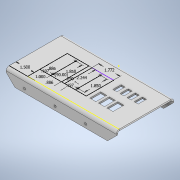
# Autodesk Inventor part: sheetmetalrightside
Saved by Autodesk Inventor 2020.2 (Build 242310000, 310)
## iProperties
Created: 2020-02-05
Part Number: sheetmetalrightside
Material: Generic
Document SubType Name: Sheet Metal
Designer: ColinP
Density: 1 g/cm^3
Sheet Metal Rule: Default
Appearance: Default
Author: ColinP
Autodesk Inventor part; units mm, degrees
ref_plane "YZ Plane" through (0, 0, 0) normal (1, 0, 0) x (0, 1, 0)
ref_plane "XZ Plane" through (0, 0, 0) normal (0, 1, 0) x (-1, 0, 0)
ref_plane "XY Plane" through (0, 0, 0) normal (0, 0, 1) x (1, 0, 0)
sketch "Sketch1" plane through (0, 0, 0) normal (0, 0, 1) x (1, 0, 0)
  line L0 (114.3, 63.5) -> (-114.3, 63.5)
  line L1 (-114.3, 63.5) -> (-114.3, -63.5)
  line L2 (-114.3, -63.5) -> (114.3, -63.5)
  line L3 (114.3, -63.5) -> (114.3, 63.5)
  point P0 (0, 0)
  dimension "d0" = 228.6
  dimension "d1" = 127
  measures "d0" distance of L2.end L1.end
  measures "d1" distance of L1.end L0.end
extrude "Plate1" add sketch "Sketch1" along normal blind 3.048
sketch "Sketch2" plane through (0, 0, 3.048) normal (0, 0, 1) x (1, 0, 0)
  line L0 (114.3, 63.5) -> (-114.3, 63.5)
  line L1 (-114.3, 63.5) -> (-96.3395, 81.4605)
  line L2 (-114.3, 63.5) -> (-88.9, 63.5) construction
  line L3 (114.3, 63.5) -> (96.3395, 81.4605)
  line L4 (114.3, 63.5) -> (139.7, 63.5) construction
  line L5 (96.3395, 81.4605) -> (-96.3395, 81.4605)
  line L6 (-114.3, 63.5) -> (-114.3, -63.5)
  line L7 (-114.3, -63.5) -> (-96.3395, -81.4605)
  line L8 (-114.3, -63.5) -> (-88.9, -63.5) construction
  line L9 (-96.3395, -81.4605) -> (96.3395, -81.4605)
  line L10 (-114.3, -63.5) -> (114.3, -63.5)
  line L11 (96.3395, -81.4605) -> (114.3, -63.5)
  point P0 (0, 0)
  dimension "d3" = 25.4
  dimension "d4" = 45
  dimension "d5" = 25.4
  dimension "d6" = 135
  dimension "d7" = 25.4
  dimension "d8" = 45
  measures "d3" distance of L0.end L1.end
  measures "d4" angle of L2 L1
  measures "d5" distance of L0.start L3.end
  measures "d6" angle of L4 L3
  measures "d7" distance of L6.end L7.end
  measures "d8" angle of L7 L8
sheet face with bend "Face2" sketch "Sketch2" thickness 3.048 toward (0, 0, -1) bend radius 3.048 relief straight relief width 3.048 relief depth 1.524
bend "Bend1"
sketch "Sketch3" plane through (0, 0, 3.048) normal (0, 0, 1) x (1, 0, 0)
  line L0 (-114.3, 63.5) -> (-114.3, -63.5) projected
  line L1 (-114.3, 63.5) -> (-114.3, 57.15)
  line L2 (-114.3, 57.15) -> (114.3, 57.15)
  line L3 (114.3, 63.5) -> (114.3, -63.5) projected
  line L4 (114.3, -63.5) -> (114.3, -57.15)
  line L5 (114.3, -57.15) -> (-114.3, -57.15)
  point P0 (0, 0)
  dimension "d14" = 6.35
  dimension "d15" = 6.35
  constraints: 8 end point, 4 point on line, 2 perpendicular
  measures "d14" distance of L0.start L1.end
  measures "d15" distance of L3.end L4.end
fold "Fold1" angle 90 bend radius 3.048 thickness 3.048 k factor 0.44 line from (-114.3, 57.15, 3.048) to (114.3, 57.15, 3.048) line at bend centre moving side (0, 1, 0) folds toward (0, 0, 1)
sketch "Sketch4" plane through (0, 0, 3.048) normal (0, 0, 1) x (1, 0, 0)
  line L0 (-114.3, -63.5) -> (-114.3, 53.7028) projected
  line L1 (-114.3, -63.5) -> (-114.3, -57.15)
  line L2 (-114.3, -57.15) -> (114.3, -57.15)
  line L3 (114.3, -63.5) -> (114.3, 53.7028) projected
  point P0 (0, 0)
  dimension "d22" = 6.35
  constraints: 4 end point, 2 point on line, 1 perpendicular
  measures "d22" distance of L0.start L1.end
fold "Fold2" angle 90 bend radius 3.048 thickness 3.048 k factor 0.44 line from (-114.3, -57.15, 3.048) to (114.3, -57.15, 3.048) line at bend centre moving side (0, 1, 0) folds toward (0, 0, 1)
sketch "Sketch5" plane through (-114.3, -54.5012, 113.5016) normal (0, 1, 0) x (1, 0, 0)
  line L0 (0, 0) -> (228.6, 0) projected
  line L1 (228.6, 0) -> (190.5, 0)
  line L2 (190.5, 0) -> (190.5, 25.4)
  line L3 (190.5, 25.4) -> (190.5, 48.006)
  line L4 (190.5, 48.006) -> (177.8, 48.006)
  line L5 (177.8, 48.006) -> (177.8, 25.4)
  line L6 (177.8, 25.4) -> (190.5, 25.4)
  line L7 (177.8, 48.006) -> (172.72, 48.006)
  line L8 (172.72, 48.006) -> (160.02, 48.006)
  line L9 (160.02, 48.006) -> (160.02, 25.4)
  line L10 (160.02, 25.4) -> (172.72, 25.4)
  line L11 (172.72, 25.4) -> (172.72, 48.006)
  line L12 (160.02, 48.006) -> (154.94, 48.006)
  line L13 (154.94, 48.006) -> (154.94, 25.4)
  line L14 (154.94, 25.4) -> (142.24, 25.4)
  line L15 (142.24, 25.4) -> (142.24, 48.006)
  line L16 (142.24, 48.006) -> (154.94, 48.006)
  line L17 (203.2, 107.4056) -> (203.2, 82.0056)
  line L18 (203.2, 107.4056) -> (228.6, 107.4056) construction
  line L19 (203.2, 82.0056) -> (194.818, 82.0056)
  line L20 (194.818, 82.0056) -> (194.818, 64.9876)
  line L21 (194.818, 64.9876) -> (203.2, 64.9876)
  line L22 (203.2, 64.9876) -> (203.2, 82.0056)
  line L23 (194.818, 82.0056) -> (188.468, 82.0056)
  line L24 (188.468, 82.0056) -> (180.086, 82.0056)
  line L25 (180.086, 82.0056) -> (180.086, 64.9876)
  line L26 (180.086, 64.9876) -> (188.468, 64.9876)
  line L27 (188.468, 64.9876) -> (188.468, 82.0056)
  line L28 (180.086, 82.0056) -> (173.736, 82.0056)
  line L29 (173.736, 82.0056) -> (173.736, 64.9876)
  line L30 (173.736, 64.9876) -> (165.354, 64.9876)
  line L31 (165.354, 64.9876) -> (165.354, 82.0056)
  line L32 (165.354, 82.0056) -> (173.736, 82.0056)
  line L33 (165.354, 82.0056) -> (159.004, 82.0056)
  line L34 (159.004, 82.0056) -> (159.004, 64.9876)
  line L35 (159.004, 64.9876) -> (150.622, 64.9876)
  line L36 (150.622, 64.9876) -> (150.622, 82.0056)
  line L37 (150.622, 82.0056) -> (159.004, 82.0056)
  line L38 (228.6, 0) -> (228.6, 107.4056) projected
  line L39 (203.2, 107.4056) -> (228.6, 107.4056)
  point P0 (114.3, 113.5016)
  dimension "d34" = 38.1
  dimension "d35" = 25.4
  dimension "d36" = 22.606
  dimension "d37" = 12.7
  dimension "d38" = 5.08
  dimension "d39" = 12.7
  dimension "d40" = 5.08
  dimension "d41" = 12.7
  dimension "d42" = 25.4
  dimension "d44" = 8.382
  dimension "d45" = 17.018
  dimension "d46" = 6.35
  dimension "d47" = 8.382
  dimension "d48" = 6.35
  dimension "d49" = 8.382
  dimension "d50" = 6.35
  dimension "d51" = 8.382
  dimension "d86" = 25.4
  constraints: 76 end point, 21 perpendicular, 14 point on line, 6 horizontal, 3 vertical, 1 collinear
  measures "d34" distance of L0.end L1.end
  measures "d35" distance of L1.end L2.end
  measures "d36" distance of L2.end L3.end
  measures "d37" distance of L3.end L4.end
  measures "d38" distance of L4.end L7.end
  measures "d39" distance of L7.end L8.end
  measures "d40" distance of L8.end L12.end
  measures "d41" distance of L13.end L14.end
  measures "d42" distance of L17.start L17.end
  measures "d44" distance of L17.end L19.end
  measures "d45" distance of L19.end L20.end
  measures "d46" distance of L19.end L23.end
  measures "d47" distance of L23.end L24.end
  measures "d48" distance of L24.end L28.end
  measures "d49" distance of L29.end L30.end
  measures "d50" distance of L31.end L33.end
  measures "d51" distance of L34.end L35.end
  measures "d86" distance of L17.start L18.end
extrude "Cut1" cut sketch "Sketch5" against normal blind 3.048
sketch "Sketch6" plane through (-114.3, -54.5012, 113.5016) normal (0, 1, 0) x (1, 0, 0)
  line L0 (0, 0) -> (228.6, 0) projected
  line L1 (0, 0) -> (38.1, 0)
  line L2 (38.1, 0) -> (38.1, 25.4)
  line L3 (38.1, 25.4) -> (60.6, 25.4)
  line L4 (60.6, 25.4) -> (83.1, 25.4)
  line L5 (83.1, 25.4) -> (83.1, 82.4)
  line L6 (83.1, 82.4) -> (38.1, 82.4)
  line L7 (38.1, 82.4) -> (38.1, 25.4)
  line L8 (60.6, 25.4) -> (60.6, 30.4)
  line L9 (60.6, 30.4) -> (60.6, 77.4)
  line L10 (83.1, 25.4) -> (89.45, 25.4)
  line L11 (89.45, 25.4) -> (89.45, 82.4)
  line L12 (89.45, 82.4) -> (134.45, 82.4)
  line L13 (134.45, 82.4) -> (134.45, 25.4)
  line L14 (134.45, 25.4) -> (89.45, 25.4)
  line L15 (111.95, 25.4) -> (111.95, 30.4)
  line L16 (111.95, 30.4) -> (111.95, 77.4)
  point P0 (114.3, 113.5016)
  dimension "d54" = 38.1
  dimension "d55" = 25.4
  dimension "d56" = 22.5
  dimension "d57" = 22.5
  dimension "d58" = 57
  dimension "d59" = 90
  dimension "d60" = 5
  dimension "d61" = 47
  dimension "d62" = 6.35
  dimension "d63" = 45
  dimension "d64" = 5
  dimension "d65" = 47
  constraints: 32 end point, 8 perpendicular, 5 point on line, 2 horizontal, 2 vertical, 1 midpoint
  measures "d54" distance of L0.start L1.end
  measures "d55" distance of L1.end L2.end
  measures "d56" distance of L2.end L3.end
  measures "d57" distance of L3.end L4.end
  measures "d58" distance of L4.end L5.end
  measures "d59" angle of L5 L4
  measures "d60" distance of L3.end L8.end
  measures "d61" distance of L8.end L9.end
  measures "d62" distance of L4.end L10.end
  measures "d63" distance of L11.end L12.end
  measures "d64" distance of L15.start L15.end
  measures "d65" distance of L15.end L16.end
hole "Hole1" at (-2.35, -54.5012, 83.1016) at (-2.35, -54.5012, 36.1016) at (-53.7, -54.5012, 36.1016) at (-53.7, -54.5012, 83.1016) direction (0, -1, 0) diameter 4.4958 depth 3.048 clearance for "Flat Head Machine Screw (82)" size "#8" standard "Ansi Unified Screw Threads"
sketch "Sketch7" plane through (96.3395, -81.4605, 119.5976) normal (0, 0, -1) x (-1, 0, 0)
  line L0 (-17.9605, 17.9605) -> (-17.9605, 20.8633) projected
  line L1 (-17.9605, 17.9605) -> (-17.9605, 7.8005)
  line L2 (-17.9605, 7.8005) -> (210.6395, 7.8005)
  line L3 (-17.9605, 7.8005) -> (45.5395, 7.8005)
  line L4 (45.5395, 7.8005) -> (109.0395, 7.8005)
  line L5 (109.0395, 7.8005) -> (172.5395, 7.8005)
  point P0 (96.3395, 81.4605)
  dimension "d73" = 10.16
  dimension "d74" = 228.6
  dimension "d75" = 90
  dimension "d76" = 63.5
  dimension "d77" = 63.5
  dimension "d78" = 63.5
  constraints: 10 end point, 3 point on line, 1 perpendicular, 1 vertical
  measures "d73" distance of L0.start L1.end
  measures "d74" distance of L1.end L2.end
  measures "d75" angle of L2 L1
  measures "d76" distance of L1.end L3.end
  measures "d77" distance of L3.end L4.end
  measures "d78" distance of L4.end L5.end
hole "Hole2" at (50.8, -73.66, 119.5976) at (-12.7, -73.66, 119.5976) at (-76.2, -73.66, 119.5976) direction (0, 0, -1) diameter 4.4958 depth 3.048 clearance for "Flat Head Machine Screw (82)" size "#8" standard "Ansi Unified Screw Threads"
equation "\"d2\" = Thickness"
equation "\"d16\" = BendReliefWidth"
equation "\"d17\" = BendReliefDepth"
equation "\"d18\" = MinimumRemnant"
equation "\"d19\" = TransitionRadius"
equation "\"d21\" = BendRadius"
equation "\"d23\" = BendReliefWidth"
equation "\"d24\" = BendReliefDepth"
equation "\"d25\" = MinimumRemnant"
equation "\"d26\" = TransitionRadius"
equation "\"d28\" = BendRadius"
equation "\"d52\" = Thickness"
equation "\"d71\" = Thickness"
equation "\"d84\" = Thickness"
equation "\"d9\" = BendRadius"
equation "\"d10\" = BendReliefWidth"
equation "\"d12\" = MinimumRemnant"
equation "\"d11\" = BendReliefDepth"
equation "\"d13\" = TransitionRadius"
equation "\"BendRadius\" = Thickness"
equation "\"BendReliefWidth\" = Thickness"
equation "\"BendReliefDepth\" = 0.5 * Thickness"
equation "\"CornerReliefSize\" = 4 * Thickness"
equation "\"MinimumRemnant\" = 2 * Thickness"
equation "\"TransitionRadius\" = BendRadius"
equation "\"JacobiRadiusSize\" = BendRadius"
equation "\"GapSize\" = Thickness"
equation "\"Thickness\" = 3.048"
body "Solid1"
